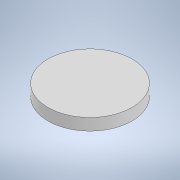
# Autodesk Inventor part: Battery
Saved by Autodesk Inventor 2022 (Build 260153000, 153)
## iProperties
Created: 2022-06-20
Part Number: Battery
Material: Generic
Document SubType Name: Modeling
Designer: Mike
Density: 1 g/cm^3
Appearance: Default
Author: Mike
Autodesk Inventor part; units mm, degrees
ref_plane "YZ Plane" through (0, 0, 0) normal (1, 0, 0) x (0, 1, 0)
ref_plane "XZ Plane" through (0, 0, 0) normal (0, 1, 0) x (-1, 0, 0)
ref_plane "XY Plane" through (0, 0, 0) normal (0, 0, 1) x (1, 0, 0)
sketch "Sketch1" plane through (0, 0, 0) normal (0, 1, 0) x (-1, 0, 0)
  circle A0 centre (0, 0) radius 25
  line L0 (8, 21) -> (8, -21)
  line L1 (8, -21) -> (-12, -21)
  line L2 (-12, -21) -> (-12, 21)
  line L3 (-12, 21) -> (8, 21)
  line L4 (8, 10) -> (20, 10)
  line L5 (20, 10) -> (20, -10)
  line L6 (20, -10) -> (8, -10)
  dimension "d0" = 50
  dimension "d1" = 20
  dimension "d2" = 20
  dimension "d3" = 42
  dimension "d4" = 21
  dimension "d5" = 10
  dimension "d6" = 8
  dimension "d7" = 20
  constraints: 14 end point, 5 perpendicular, 2 point on line, 1 centre point, 1 coincident, 1 horizontal, 1 vertical
  measures "d0" diameter of A0
  measures "d1" distance between parallel lines of L6 L4
  measures "d2" distance between parallel lines of L2 L0
  measures "d3" distance between parallel lines of L1 L3
  measures "d4" distance from line of L1 point (0, 0)
  measures "d5" distance from line of L4 point (0, 0)
  measures "d6" distance from line of L0 point (0, 0)
  measures "d7" distance from line of L5 point (0, 0)
extrude "Extrusion1" add sketch "Sketch1" along normal blind 2 contours A0 | L0 L1 L2 L3 | L4 L5 L6 L0
extrude "Extrusion2" add sketch "Sketch1" against normal blind 5
body "Solid1"
